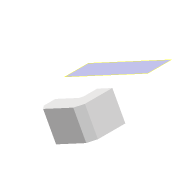
# Autodesk Inventor part: Matchboxscope_Lightperiscope_V0
Saved by Autodesk Inventor 2022 (Build 260153000, 153)
## iProperties
Created: 2022-03-26
Part Number: Matchboxscope_Lightperiscope_V0
Material: Generic
Document SubType Name: Modeling
Designer: Prakash Lab
Density: 1 g/cm^3
Appearance: Default
Author: Prakash Lab
Autodesk Inventor part; units mm, degrees
ref_plane "YZ Plane" through (0, 0, 0) normal (1, 0, 0) x (0, 1, 0)
ref_plane "XZ Plane" through (0, 0, 0) normal (0, 1, 0) x (-1, 0, 0)
ref_plane "XY Plane" through (0, 0, 0) normal (0, 0, 1) x (1, 0, 0)
ref_plane "Work Plane1" through (118.9518, 9.9874, -13.1749) normal (0.4728584, -0.8811384, 0) x (0, 0, -1)
sketch "Sketch1" plane through (118.9518, 9.9874, -13.1749) normal (0.4728584, -0.8811384, 0) x (0, 0, -1)
  line L0 (-0.7641, 6) -> (-0.7641, -6)
  line L1 (-16.5984, 5.4988) -> (-16.5984, 6)
  line L2 (-7.5984, -7.7203) -> (-5.5984, -7.7203)
  line L3 (-7.5984, -21.1989) -> (-0.5984, -21.1989)
  line L4 (-1.2281, -14.4596) -> (-31.7652, -14.4596) construction
  line L5 (-16.5984, 11.5008) -> (-16.5984, -0.9971) projected
  line L6 (-15.5984, -2) -> (-12.5984, -2)
  line L7 (-16.5984, 2) -> (-12.5984, 2)
  line L8 (-16.5984, -3.8894) -> (-24.0984, -3.8894)
  line L9 (-24.0984, -3.8894) -> (-25.5984, -5.3894)
  line L10 (-25.5984, -5.3894) -> (-25.5984, -8.4596)
  line L11 (-25.5984, -8.4596) -> (-25.5984, -20.4596)
  line L12 (-25.5984, -20.4596) -> (-32.0984, -20.4596)
  line L13 (-32.0984, -20.4596) -> (-35.5984, -16.9596)
  line L14 (-35.5984, -16.9596) -> (-35.5984, 2.37)
  line L15 (-35.5984, 2.37) -> (-32.0984, 5.87)
  line L16 (-32.0984, 5.87) -> (-16.5984, 5.87)
  line L17 (-16.5984, 0.8574) -> (-16.5984, 5.87)
  line L18 (-16.5984, 2.1106) -> (-43.439, 2.1106) construction
  line L19 (-16.5984, -0.9971) -> (-16.5984, -3.8894)
  point P0 (-13.1749, -109.5356)
  point P1 (-16.5984, 0.8574)
  dimension "d22" = 13.4786
  dimension "d23" = 6.7393
  dimension "d25" = 135
  dimension "d26" = 4
  dimension "d27" = 6
  dimension "d28" = 3.7594
  dimension "d29" = 6
  dimension "d31" = 10
  dimension "d37" = 3.5
  dimension "d38" = 3.5
  dimension "d40" = 1.5
  dimension "d42" = 19
  constraints: 38 end point, 7 horizontal, 4 perpendicular, 3 collinear, 3 point on line, 2 parallel, 10 other
  measures "d22" distance between parallel lines of L2 L3
  measures "d23" distance between parallel lines of L3 L4
  measures "d25" angle of L12 L13
  measures "d26" distance between parallel lines of L7 L6
  measures "d27" distance between parallel lines of L8 L18
  measures "d28" distance between parallel lines of L16 L18
  measures "d29" distance between parallel lines of L12 L4
  measures "d31" distance between parallel lines of L10 L14
  measures "d37" horizontal distance of L12.end L13.end
  measures "d38" horizontal distance of L15.end L14.end
  measures "d40" horizontal distance of L8.end L9.end
  measures "d42" distance between parallel lines of L19 L14
extrude "Extrusion1" add sketch "Sketch1" along normal blind 1.5
sketch "Sketch2" plane through (119.6611, 8.6657, -13.1749) normal (0.4728584, -0.8811384, 0) x (0.8811384, 0.4728584, 0)
  line L0 (2.37, 35.5984) -> (-16.9596, 35.5984) projected
  line L1 (-16.9596, 35.5984) -> (-20.4596, 32.0984) projected
  line L2 (-20.4596, 32.0984) -> (-20.4596, 25.5984) projected
  line L3 (-20.4596, 25.5984) -> (-5.3894, 25.5984) projected
  line L4 (-5.3894, 25.5984) -> (-3.8894, 24.0984) projected
  line L5 (-3.8894, 24.0984) -> (-3.8894, 16.5984) projected
  line L6 (5.87, 16.5984) -> (5.87, 32.0984) projected
  line L7 (5.87, 32.0984) -> (2.37, 35.5984) projected
  line L8 (-3.8894, 16.5984) -> (5.87, 16.5984) projected
  line L9 (-16.3383, 34.0984) -> (1.7487, 34.0984)
  line L10 (1.7487, 34.0984) -> (4.37, 31.4771)
  line L11 (4.37, 31.4771) -> (4.37, 18.0984)
  line L12 (4.37, 18.0984) -> (-0.9902, 18.0984)
  line L13 (-0.9902, 18.0984) -> (-2.3894, 18.1112)
  line L14 (-2.3894, 18.1112) -> (-2.3894, 24.7197)
  line L15 (-2.3894, 24.7197) -> (-4.7681, 27.0984)
  line L16 (-4.7681, 27.0984) -> (-8.9884, 27.0984)
  line L17 (-8.9884, 27.0984) -> (-9.9596, 27.0984)
  line L18 (-9.9596, 27.0984) -> (-18.9596, 27.0984)
  line L19 (-18.9596, 27.0984) -> (-18.9596, 31.4771)
  line L20 (-18.9596, 31.4771) -> (-16.3383, 34.0984)
  point P0 (-109.5356, 13.1749)
  dimension "d41" = 1.5
  constraints: 24 end point, 1 horizontal, 6 other
  measures "d41" distance between parallel lines of L0 L9
extrude "Extrusion2" add sketch "Sketch2" along normal blind 14
sketch "Sketch3" plane through (103.7391, 1.8236, 12.4235) normal (0, 0, -1) x (-0.8811384, -0.4728584, 0)
  circle A0 centre (-2.8052, -7.75) radius 4.5
  line L0 (3.1948, 0) -> (-8.8052, 0) projected
  line L1 (-8.8052, 0) -> (-8.8052, -15.5) projected
  line L2 (3.1948, -15.5) -> (-8.8052, -15.5) projected
  line L3 (3.1948, 0) -> (3.1948, -15.5) projected
  point P0 (92.2708, 47.4471)
  constraints: 1 centre point
extrude "Extrusion3" cut sketch "Sketch3" against normal blind 1.5 contours A0
sketch "Sketch8" plane through (119.6748, 8.673, 3.4235) normal (0, 0, 1) x (0.8811384, 0.4728584, 0)
  circle A0 centre (-19.1075, 3.6497) radius 1.4001 projected
  circle A1 centre (-14.1578, 7.8923) radius 2 projected
  circle A2 centre (-14.1578, 7.8923) radius 3.3708
  point P0 (-109.5511, 48.9471)
  constraints: 1 centre point
extrude "Extrusion8" cut sketch "Sketch8" along normal mid plane 14 contours A1 | A2
sketch "Sketch9" plane through (118.7885, 8.1974, 4.9235) normal (0, 0, 1) x (0.8811384, 0.4728584, 0)
  circle A0 centre (0.9902, -6.25) radius 1.352 projected
  circle A1 centre (0.9902, -6.25) radius 2.6601
  point P0 (-108.5454, 48.9471)
  constraints: 1 centre point, 1 coincident
extrude "Extrusion9" cut sketch "Sketch9" along normal mid plane 14 contours A0 | A1
equation "\"d23\" = 0.5 * d22"
body "Solid1"
